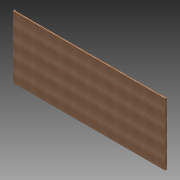
# Autodesk Inventor part: Base
Saved by Autodesk Inventor 2014 SP1 (Build 180222100, 222)
## iProperties
Created: 2015-03-28
Part Number: Base
Material: Wood (Birch)
Document SubType Name: Modeling
Designer: tuleu
Density: 0.55 g/cm^3
Appearance: Birch - Natural Polished
Author: tuleu
Autodesk Inventor part; units mm, degrees
ref_plane "YZ Plane" through (0, 0, 0) normal (1, 0, 0) x (0, 1, 0)
ref_plane "XZ Plane" through (0, 0, 0) normal (0, 1, 0) x (-1, 0, 0)
ref_plane "XY Plane" through (0, 0, 0) normal (0, 0, 1) x (1, 0, 0)
sketch "Sketch1" plane through (0, 0, 0) normal (0, 1, 0) x (-1, 0, 0)
  line L0 (1400, 575) -> (-1400, 575)
  line L1 (-1400, 575) -> (-1400, -575)
  line L2 (-1400, -575) -> (1400, -575)
  line L3 (1400, -575) -> (1400, 575)
  line L4 (0, -575) -> (0, 575)
  line L5 (-1400, 0) -> (1400, 0)
  point P0 (0, 0)
  dimension "d0" = 2800
  dimension "d1" = 1150
  constraints: 12 end point, 6 midpoint, 2 parallel, 1 horizontal, 1 perpendicular
  measures "d0" distance of L1.end L2.end
  measures "d1" distance of L2.end L0.start
extrude "Extrusion1" add sketch "Sketch1" along normal blind 19
sketch "Sketch2" plane through (0, 19, 0) normal (0, 1, 0) x (1, 0, 0)
  line L0 (1400, 575) -> (-1400, 575) projected
  line L1 (-1400, 575) -> (-1400, -575) projected
  line L2 (-1400, -575) -> (1400, -575) projected
  line L3 (1400, -575) -> (1400, 575) projected
  line L4 (-1385, -575) -> (-1385, 575)
  line L5 (1385, 575) -> (1385, -575)
  line L6 (-1385, -575) -> (-1400, -575)
  line L7 (-1400, 575) -> (-1400, -575)
  line L8 (1400, 575) -> (1400, -575)
  line L9 (1400, -575) -> (1385, -575)
  line L10 (-1400, 575) -> (-1385, 575)
  line L11 (1385, 575) -> (1400, 575)
  point P0 (0, 0)
  dimension "d4" = 15
  dimension "d5" = 15
  constraints: 16 end point, 4 perpendicular, 3 collinear, 2 point on line, 1 parallel
  measures "d4" distance between parallel lines of L1 L4
  measures "d5" distance between parallel lines of L3 L5
extrude "Extrusion2" add sketch "Sketch2" along normal blind 19 contours L3 L2 L5 L0 | L4 L2 L1 L0
sketch "Sketch4" plane through (0, 19, 0) normal (0, 1, 0) x (1, 0, 0)
  line L0 (-1385, 575) -> (-1385, -575) projected
  line L1 (-1385, -575) -> (1385, -575) projected
  line L2 (1385, -575) -> (1385, 575) projected
  line L3 (1385, 575) -> (-1385, 575) projected
  line L4 (-1255, -225) -> (-1309.8, -225) projected
  line L5 (-1177.5, 175) -> (-1232.3, 175) projected
  line L6 (-1275, 475) -> (-1385, 475) projected
  line L7 (-1165, 475) -> (-1270, 475) projected
  line L8 (-1060, 475) -> (-1160, 475) projected
  line L9 (-950, 475) -> (-1055, 475) projected
  line L10 (-835, 475) -> (-945, 475) projected
  line L11 (-735, 475) -> (-830, 475) projected
  line L12 (-625, 475) -> (-730, 475) projected
  line L13 (-520, 475) -> (-620, 475) projected
  line L14 (-410, 475) -> (-515, 475) projected
  line L15 (-305, 475) -> (-405, 475) projected
  line L16 (-195, 475) -> (-300, 475) projected
  line L17 (-95, 475) -> (-190, 475) projected
  line L18 (20, 475) -> (-90, 475) projected
  line L19 (130, 475) -> (25, 475) projected
  line L20 (235, 475) -> (135, 475) projected
  line L21 (345, 475) -> (240, 475) projected
  line L22 (460, 475) -> (350, 475) projected
  line L23 (560, 475) -> (465, 475) projected
  line L24 (670, 475) -> (565, 475) projected
  line L25 (775, 475) -> (675, 475) projected
  line L26 (885, 475) -> (780, 475) projected
  line L27 (990, 475) -> (890, 475) projected
  line L28 (1100, 475) -> (995, 475) projected
  line L29 (1200, 475) -> (1105, 475) projected
  line L30 (1385, 475) -> (1205, 475) projected
  line L31 (0, 575) -> (0, 475)
  line L32 (-1385, 525) -> (1385, 525)
  line L33 (-1332.5, 542.5) -> (1297.5, 542.5)
  line L34 (-1330, 475) -> (-1330, -575)
  line L35 (-1217.5, 475) -> (-1217.5, -575)
  line L36 (-1110, 475) -> (-1110, -575)
  line L37 (-1002.5, 475) -> (-1002.5, -575)
  line L38 (-890, 475) -> (-890, -575)
  line L39 (-782.5, 475) -> (-782.5, -575)
  line L40 (-677.5, 475) -> (-677.5, -575)
  line L41 (-570, 475) -> (-570, -575)
  line L42 (-462.5, 475) -> (-462.5, -575)
  line L43 (-355, 475) -> (-355, -575)
  line L44 (-247.5, 475) -> (-247.5, -575)
  line L45 (-142.5, 475) -> (-142.5, -575)
  line L46 (-35, 475) -> (-35, -575)
  line L47 (77.5, 475) -> (77.5, -575)
  line L48 (185, 475) -> (185, -575)
  line L49 (292.5, 475) -> (292.5, -575)
  line L50 (405, 475) -> (405, -575)
  line L51 (512.5, 475) -> (512.5, -575)
  line L52 (617.5, 475) -> (617.5, -575)
  line L53 (725, 475) -> (725, -575)
  line L54 (832.5, 475) -> (832.5, -575)
  line L55 (940, 475) -> (940, -575)
  line L56 (1047.5, 475) -> (1047.5, -575)
  line L57 (1152.5, 475) -> (1152.5, -575)
  line L58 (1295, 475) -> (1295, -575)
  line L59 (-780, 507.5) -> (-780, -195)
  line L60 (-785, -205) -> (-785, 507.5)
  line L61 (-675, 507.5) -> (-675, 205)
  line L62 (-680, 205) -> (-680, 507.5)
  line L63 (-567.5, 507.5) -> (-567.5, -195)
  line L64 (10112.5717, -224.7042) -> (10045.4368, -224.5421)
  line L65 (-572.5, -195) -> (-572.5, 507.5)
  line L66 (-460, 507.5) -> (-460, 205)
  line L67 (-465, 205) -> (-465, 507.5)
  line L68 (-352.5, 507.5) -> (-352.5, -195)
  line L69 (10327.5757, -225.2236) -> (10260.4408, -225.0614)
  line L70 (-357.5, -195) -> (-357.5, 507.5)
  line L71 (-245, 507.5) -> (-245, 205)
  line L72 (-633754.4369, 240.5665) -> (-633821.572, 240.5713)
  line L73 (-250, 205) -> (-250, 507.5)
  line L74 (-140, 507.5) -> (-140, -205)
  line L75 (-145, -195) -> (-145, 507.5)
  line L76 (-1327.5, 507.5) -> (-1327.5, -195)
  line L77 (-1262.5, -205) -> (-1332.5, -205)
  line L78 (-1332.5, -205) -> (-1332.5, 542.5)
  line L79 (-1215, 507.5) -> (-1215, 205)
  line L80 (-1220, 205) -> (-1220, 507.5)
  line L81 (-1107.5, 507.5) -> (-1107.5, -195)
  line L82 (-1112.5, -195) -> (-1112.5, 507.5)
  line L83 (-1000, 507.5) -> (-1000, 205)
  line L84 (-1005, 205) -> (-1005, 507.5)
  line L85 (-887.5, 507.5) -> (-887.5, -205)
  line L86 (-887.5, -205) -> (-952.5, -205)
  line L87 (-892.5, -195) -> (-892.5, 507.5)
  line L88 (-32.5, 507.5) -> (-32.5, -195)
  line L89 (-37.5, -205) -> (-37.5, 507.5)
  line L90 (80, 507.5) -> (80, 205)
  line L91 (75, 205) -> (75, 507.5)
  line L92 (-1220, 507.5) -> (-1327.5, 507.5)
  line L93 (-1112.5, 507.5) -> (-1215, 507.5)
  line L94 (-1005, 507.5) -> (-1107.5, 507.5)
  line L95 (-892.5, 507.5) -> (-1000, 507.5)
  line L96 (-785, 507.5) -> (-887.5, 507.5)
  line L97 (-680, 507.5) -> (-780, 507.5)
  line L98 (-572.5, 507.5) -> (-675, 507.5)
  line L99 (-465, 507.5) -> (-567.5, 507.5)
  line L100 (-357.5, 507.5) -> (-460, 507.5)
  line L101 (-250, 507.5) -> (-352.5, 507.5)
  line L102 (-145, 507.5) -> (-245, 507.5)
  line L103 (-37.5, 507.5) -> (-140, 507.5)
  line L104 (75, 507.5) -> (-32.5, 507.5)
  line L105 (187.5, 507.5) -> (187.5, -195)
  line L106 (182.5, -195) -> (182.5, 507.5)
  line L107 (295, 507.5) -> (295, 205)
  line L108 (290, 205) -> (290, 507.5)
  line L109 (407.5, 507.5) -> (407.5, -205)
  line L110 (407.5, -205) -> (343.6554, -205)
  line L111 (402.5, -195) -> (402.5, 507.5)
  line L112 (515, 507.5) -> (515, -195)
  line L113 (510, -205) -> (510, 507.5)
  line L114 (620, 507.5) -> (620, 205)
  line L115 (615, 205) -> (615, 507.5)
  line L116 (727.5, 507.5) -> (727.5, -195)
  line L117 (722.5, -205) -> (722.5, 507.5)
  line L118 (835, 507.5) -> (835, 205)
  line L119 (830, 205) -> (830, 507.5)
  line L120 (942.5, 507.5) -> (942.5, -195)
  line L121 (937.5, -195) -> (937.5, 507.5)
  line L122 (1050, 507.5) -> (1050, 205)
  line L123 (1045, 205) -> (1045, 507.5)
  line L124 (1155, 507.5) -> (1155, -205)
  line L125 (1150, -195) -> (1150, 507.5)
  line L126 (182.5, 507.5) -> (80, 507.5)
  line L127 (290, 507.5) -> (187.5, 507.5)
  line L128 (402.5, 507.5) -> (295, 507.5)
  line L129 (510, 507.5) -> (407.5, 507.5)
  line L130 (615, 507.5) -> (515, 507.5)
  line L131 (722.5, 507.5) -> (620, 507.5)
  line L132 (830, 507.5) -> (727.5, 507.5)
  line L133 (937.5, 507.5) -> (835, 507.5)
  line L134 (1045, 507.5) -> (942.5, 507.5)
  line L135 (1150, 507.5) -> (1050, 507.5)
  line L136 (1292.5, 507.5) -> (1155, 507.5)
  line L137 (1297.5, 542.5) -> (1297.5, -195)
  line L138 (1292.5, -195) -> (1292.5, 507.5)
  line L139 (-1327.5, -195) -> (-1262.5, -195)
  line L140 (-1262.5, -195) -> (-1262.5, -205)
  line L141 (-1280.2, -200) -> (-1280.2, -225) projected
  line L142 (-1309.8, -250) -> (-1309.8, -200) projected
  line L143 (-1309.8, -200) -> (-1280.2, -200)
  line L144 (-1295, -200) -> (-1295, -195)
  line L145 (-1220, 205) -> (-1245, 205)
  line L146 (-1245, 205) -> (-1245, 195)
  line L147 (-1215, 205) -> (-1190, 205)
  line L148 (-1190, 205) -> (-1190, 195)
  line L149 (-1112.5, -195) -> (-1137.5, -195)
  line L150 (-1137.5, -195) -> (-1137.5, -205)
  line L151 (-1107.5, -195) -> (-1082.5, -195)
  line L152 (-1082.5, -195) -> (-1082.5, -205)
  line L153 (-1082.5, -205) -> (-1137.5, -205)
  line L154 (-1005, 205) -> (-1030, 205)
  line L155 (-1030, 205) -> (-1030, 195)
  line L156 (-1000, 205) -> (-975, 205)
  line L157 (-975, 205) -> (-975, 195)
  line L158 (-892.5, -195) -> (-952.5, -195)
  line L159 (-952.5, -195) -> (-952.5, -205)
  line L160 (-952.5, -200) -> (-952.5, -500) projected
  line L161 (-712.5, -225) -> (-712.5, -200) projected
  line L162 (-712.5, -195) -> (-712.5, -205)
  line L163 (-705, 200) -> (-705, -100) projected
  line L164 (-650, 175) -> (-650, 200) projected
  line L165 (-397.5, -200) -> (-397.5, -500) projected
  line L166 (-342.5, -225) -> (-342.5, -200) projected
  line L167 (-212.5, -200) -> (-212.5, -500) projected
  line L168 (-275, 200) -> (-275, -100) projected
  line L169 (-220, 175) -> (-220, 200) projected
  line L170 (27.5, -225) -> (27.5, -200) projected
  line L171 (50, 200) -> (50, -100) projected
  line L172 (105, 175) -> (105, 200) projected
  line L173 (265, 200) -> (265, -100) projected
  line L174 (320, 175) -> (320, 200) projected
  line L175 (157.5, -200) -> (157.5, -500) projected
  line L176 (212.5, -225) -> (212.5, -200) projected
  line L177 (-680, 205) -> (-705, 205)
  line L178 (-705, 205) -> (-705, 195)
  line L179 (-650, 205) -> (-650, 195)
  line L180 (-582.5, -200) -> (-582.5, -500) projected
  line L181 (-527.5, -225) -> (-527.5, -200) projected
  line L182 (-572.5, -195) -> (-582.5, -195)
  line L183 (-582.5, -195) -> (-582.5, -205)
  line L184 (-567.5, -195) -> (-527.5, -195)
  line L185 (-527.5, -195) -> (-527.5, -205)
  line L186 (-490, 200) -> (-490, -100) projected
  line L187 (-435, 175) -> (-435, 200) projected
  line L188 (342.5, -200) -> (342.5, -500) projected
  line L189 (582.5, -225) -> (582.5, -200) projected
  line L190 (590, 200) -> (590, -100) projected
  line L191 (645, 175) -> (645, 200) projected
  line L192 (712.5, -200) -> (712.5, -500) projected
  line L193 (767.5, -225) -> (767.5, -200) projected
  line L194 (897.5, -200) -> (897.5, -500) projected
  line L195 (952.5, -225) -> (952.5, -200) projected
  line L196 (805, 200) -> (805, -100) projected
  line L197 (860, 175) -> (860, 200) projected
  line L198 (1020, 200) -> (1020, -100) projected
  line L199 (1075, 175) -> (1075, 200) projected
  line L200 (1082.5, -200) -> (1082.5, -500) projected
  line L201 (1267.5, -200) -> (1267.5, -500) projected
  line L202 (1322.5, -225) -> (1322.5, -200) projected
  line L203 (-397.5, -205) -> (-397.5, -195)
  line L204 (-397.5, -195) -> (-357.5, -195)
  line L205 (-352.5, -195) -> (-342.5, -195)
  line L206 (-342.5, -195) -> (-342.5, -205)
  line L207 (-212.5, -195) -> (-212.5, -205)
  line L208 (-465, 205) -> (-490, 205)
  line L209 (-490, 205) -> (-490, 195)
  line L210 (-460, 205) -> (-435, 205)
  line L211 (-435, 205) -> (-435, 195)
  line L212 (-275, 205) -> (-275, 195)
  line L213 (-220, 205) -> (-245, 205)
  line L214 (-220, 205) -> (-220, 195)
  line L215 (75, 205) -> (50, 205)
  line L216 (50, 205) -> (50, 195)
  line L217 (105, 195) -> (105, 205)
  line L218 (105, 205) -> (80, 205)
  line L219 (290, 205) -> (265, 205)
  line L220 (265, 205) -> (265, 195)
  line L221 (320, 195) -> (320, 205)
  line L222 (320, 205) -> (295, 205)
  line L223 (620, 205) -> (645, 205)
  line L224 (645, 205) -> (645, 195)
  line L225 (590, 195) -> (590, 205)
  line L226 (590, 205) -> (615, 205)
  line L227 (805, 205) -> (805, 195)
  line L228 (860, 195) -> (860, 205)
  line L229 (1020, 195) -> (1020, 205)
  line L230 (1045, 205) -> (1020, 205)
  line L231 (1050, 205) -> (1075, 205)
  line L232 (1075, 205) -> (1075, 195)
  line L233 (27.5, -195) -> (27.5, -205)
  line L234 (27.5, -205) -> (27.5075, -205)
  line L235 (182.5, -195) -> (157.5, -195)
  line L236 (157.5, -195) -> (157.5, -205)
  line L237 (212.5, -205) -> (212.5, -195)
  line L238 (212.5, -195) -> (187.5, -195)
  line L239 (402.5, -195) -> (342.5, -195)
  line L240 (342.5, -195) -> (342.5, -205)
  line L241 (342.5, -205) -> (343.6554, -205)
  line L242 (515, -195) -> (582.5, -195)
  line L243 (582.5, -195) -> (582.5, -205)
  line L244 (727.5, -195) -> (767.5, -195)
  line L245 (767.5, -205) -> (767.5, -195)
  line L246 (937.5, -195) -> (897.5, -195)
  line L247 (897.5, -205) -> (897.5, -195)
  line L248 (952.5, -205) -> (952.5, -195)
  line L249 (952.5, -195) -> (942.5, -195)
  line L250 (1150, -195) -> (1082.5, -195)
  line L251 (1082.5, -195) -> (1082.5, -205)
  line L252 (1292.5, -195) -> (1267.5, -195)
  line L253 (1267.5, -195) -> (1267.5, -205)
  line L254 (1297.5, -195) -> (1322.5, -195)
  line L255 (1322.5, -195) -> (1322.5, -205)
  line L256 (-785, -205) -> (-712.5, -205)
  line L257 (-780, -195) -> (-712.5, -195)
  line L258 (-527.5, -205) -> (-582.5, -205)
  line L259 (-397.5, -205) -> (-342.5, -205)
  line L260 (-212.5, -195) -> (-145, -195)
  line L261 (-212.5, -205) -> (-140, -205)
  line L262 (27.5, -195) -> (-32.5, -195)
  line L263 (-37.5, -205) -> (27.5, -205)
  line L264 (157.5, -205) -> (212.5, -205)
  line L265 (722.5, -205) -> (767.5, -205)
  line L266 (952.5, -205) -> (897.5, -205)
  line L267 (1082.5, -205) -> (1155, -205)
  line L268 (1267.5, -205) -> (1322.5, -205)
  line L269 (510, -205) -> (582.5, -205)
  line L270 (-1245, 195) -> (-1190, 195)
  line L271 (-1030, 195) -> (-975, 195)
  line L272 (-675, 205) -> (-650, 205)
  line L273 (-650, 195) -> (-705, 195)
  line L274 (-490, 195) -> (-435, 195)
  line L275 (-275, 205) -> (-250, 205)
  line L276 (-275, 195) -> (-220, 195)
  line L277 (105, 195) -> (50, 195)
  line L278 (265, 195) -> (320, 195)
  line L279 (645, 195) -> (590, 195)
  line L280 (805, 195) -> (860, 195)
  line L281 (1020, 195) -> (1075, 195)
  line L282 (-1232.3, 200) -> (-1245, 200) construction
  line L283 (830, 205) -> (805, 205)
  line L284 (835, 205) -> (860, 205)
  point P0 (0, 0)
  point P1 (0, 525)
  point P2 (1385, -205)
  point P3 (-1385, 195)
  dimension "d12" = 35
  dimension "d13" = 5
  dimension "d18" = 5
  dimension "d19" = 55
  dimension "d20" = 5
  dimension "d21" = 5
  dimension "d22" = 5
  dimension "d23" = 5
  dimension "d24" = 5
  dimension "d25" = 5
  dimension "d26" = 5
  dimension "d27" = 5
  dimension "d28" = 5
  dimension "d29" = 5
  dimension "d30" = 5
  dimension "d31" = 5
  dimension "d32" = 5
  dimension "d33" = 5
  dimension "d34" = 5
  dimension "d35" = 5
  dimension "d36" = 5
  dimension "d37" = 5
  dimension "d38" = 5
  dimension "d39" = 5
  dimension "d40" = 5
  dimension "d41" = 5
  dimension "d42" = 5
  dimension "d43" = 10
  constraints: 433 end point, 123 collinear, 63 parallel, 40 perpendicular, 30 midpoint, 19 vertical, 16 equal length, 12 horizontal, 5 point on line, 58 other
  measures "d12" distance between parallel lines of L92 L33
  measures "d13" distance between parallel lines of L78 L76
  measures "d18" distance between parallel lines of L79 L80
  measures "d19" distance between parallel lines of L146 L148
  measures "d20" distance between parallel lines of L81 L82
  measures "d21" distance between parallel lines of L83 L84
  measures "d22" distance between parallel lines of L85 L87
  measures "d23" distance between parallel lines of L59 L60
  measures "d24" distance between parallel lines of L62 L61
  measures "d25" distance between parallel lines of L63 L65
  measures "d26" distance between parallel lines of L66 L67
  measures "d27" distance between parallel lines of L70 L68
  measures "d28" distance between parallel lines of L74 L75
  measures "d29" distance between parallel lines of L71 L73
  measures "d30" distance between parallel lines of L88 L89
  measures "d31" distance between parallel lines of L90 L91
  measures "d32" distance between parallel lines of L107 L108
  measures "d33" distance between parallel lines of L114 L115
  measures "d34" distance between parallel lines of L118 L119
  measures "d35" distance between parallel lines of L123 L122
  measures "d36" distance between parallel lines of L105 L106
  measures "d37" distance between parallel lines of L109 L111
  measures "d38" distance between parallel lines of L112 L113
  measures "d39" distance between parallel lines of L116 L117
  measures "d40" distance between parallel lines of L120 L121
  measures "d41" distance between parallel lines of L124 L125
  measures "d42" distance between parallel lines of L137 L138
  measures "d43" distance between parallel lines of L270 L145
extrude "Extrusion3" cut sketch "Sketch4" against normal blind 1.5 contours L78 L33 L31 L32 | L32 L31 L104 L88 L18 L89 L103 L74 L17 L75 L102 L71 L16 L73 L101 L68 L15 L70 L100 L66 L14 L67 L99 L63 L13 L65 L98 L61 L12 L62 L97 L59 L11 L60 L96 L85 L10 L87 L95 L83 L9 L84 L94 L81 L8 L82 L93 L79 L7 L80 L92 L76 L6 L78 | L33 L137 L32 L31 | L6 L34 L77 L78 | L32 L137 L30 L138 L136 L124 L29 L125 L135 L122 L28 L123 L134 L120 L27 L121 L133 L118 L26 L119 L132 L116 L25 L117 L131 L114 L24 L115 L130 L112 L23 L113 L129 L109 L22 L111 L128 L107 L21 L108 L127 L105 L20 L106 L126 L90 L19 L91 L104 L31 | L6 L76 L139 L144 L143 L142 L77 L34 | L137 L254 L255 L202 L268 L58 L30 | L142 L143 L141 L77 | L88 L262 L233 L170 L263 L46 L18 | L19 L47 L277 L171 L216 L215 L91 | L58 L268 L201 L253 L252 L138 L30 | L153 L150 L149 L82 L8 L36 | L36 L8 L81 L151 L152 L153 | L270 L146 L145 L80 L7 L35 | L35 L7 L79 L147 L148 L270 | L141 L143 L144 L139 L140 L77 | L46 L263 L89 L18 | L19 L90 L218 L217 L172 L277 L47 | L271 L155 L154 L84 L9 L37 | L37 L9 L83 L156 L157 L271 | L267 L200 L251 L250 L125 L29 L57 | L57 L29 L124 L267 | L86 L159 L158 L87 L10 L38 | L38 L10 L85 L86 | L281 L198 L229 L230 L123 L28 L56 | L56 L28 L122 L231 L232 L199 L281 | L256 L60 L11 L39 | L39 L11 L59 L257 L162 L161 L256 | L266 L194 L247 L246 L121 L27 L55 | L55 L27 L120 L249 L248 L195 L266 | L273 L163 L178 L177 L62 L12 L40 | L40 L12 L61 L272 L179 L164 L273 | L74 L261 L45 L17 | L261 L167 L207 L260 L75 L17 L45 | L20 L48 L264 L175 L236 L235 L106 | L48 L20 L105 L238 L237 L176 L264 | L280 L196 L227 L283 L119 L26 L54 | L54 L26 L118 L284 L228 L197 L280 | L258 L180 L183 L182 L65 L13 L41 | L41 L13 L63 L184 L185 L181 L258 | L276 L168 L212 L275 L73 L16 L44 | L44 L16 L71 L213 L214 L169 L276 | L278 L173 L220 L219 L108 L21 L49 | L49 L21 L107 L222 L221 L174 L278 | L265 L117 L25 L53 | L53 L25 L116 L244 L245 L193 L265 | L274 L186 L209 L208 L67 L14 L42 | L42 L14 L66 L210 L211 L187 L274 | L259 L165 L203 L204 L70 L15 L43 | L43 L15 L68 L205 L206 L166 L259 | L110 L241 L188 L240 L239 L111 L22 L50 | L50 L22 L109 L110 | L279 L190 L225 L226 L115 L24 L52 | L52 L24 L114 L223 L224 L191 L279 | L269 L113 L23 L51 | L51 L23 L112 L242 L243 L189 L269
body "Solid1"
